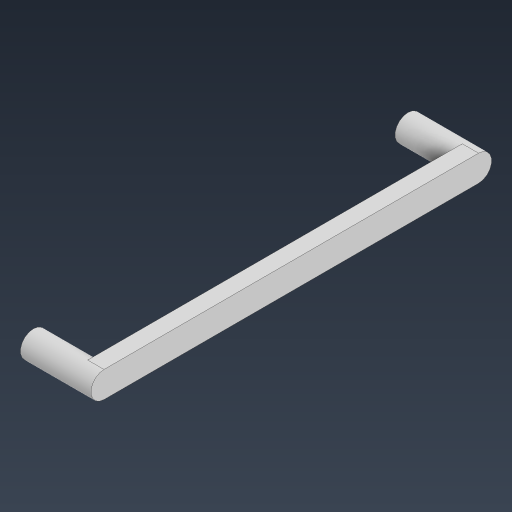
# Autodesk Inventor part: tester
Saved by Autodesk Inventor 2024 (Build 280153000, 153)
## iProperties
Created: 2025-10-03
Part Number: tester
Material: Generic
Document SubType Name: Modeling
Designer: Piter
Density: 1 g/cm^3
Appearance: Default
Author: Piter
Autodesk Inventor part; units mm, degrees
ref_plane "YZ Plane" through (0, 0, 0) normal (1, 0, 0) x (0, 1, 0)
ref_plane "XZ Plane" through (0, 0, 0) normal (0, 1, 0) x (-1, 0, 0)
ref_plane "XY Plane" through (0, 0, 0) normal (0, 0, 1) x (1, 0, 0)
sketch "Sketch2" plane through (0, 0, 0) normal (1, 0, 0) x (0, 1, 0)
  circle A0 centre (0, 0) radius 2.4
  line L0 (0, 0) -> (0, -69)
  circle A1 centre (0, -69) radius 2.4
  line L1 (2.4, 0) -> (2.4, -69)
  line L2 (-2.4, -69) -> (-2.4, 0)
  dimension "d6" = 4.8
  dimension "d13" = 69
  dimension "d14" = 4.8
  constraints: 6 end point, 4 point on circle, 2 centre point, 2 coincident, 2 vertical, 1 parallel
  measures "d6" diameter of A0
  measures "d13" distance of L0.start L0.end
  measures "d14" diameter of A1
extrude "Extrusion1" add sketch "Sketch2" along normal blind 3
extrude "Extrusion2" add sketch "Sketch2" against normal blind 10 contours A0 | A1
body "Solid1"
